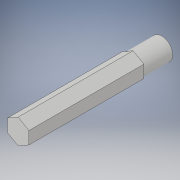
# Autodesk Inventor part: Sanded Hex Rod
Saved by Autodesk Inventor 2018 (Build 220112000, 112)
## iProperties
Created: 2019-01-13
Part Number: Sanded Hex Rod
Material: Generic
Document SubType Name: Modeling
Designer: Gabriel
Density: 1 g/cm^3
Appearance: Default
Author: Gabriel
Autodesk Inventor part; units mm, degrees
ref_plane "YZ Plane" through (0, 0, 0) normal (1, 0, 0) x (0, 1, 0)
ref_plane "XZ Plane" through (0, 0, 0) normal (0, 1, 0) x (-1, 0, 0)
ref_plane "XY Plane" through (0, 0, 0) normal (0, 0, 1) x (1, 0, 0)
sketch "Sketch1" plane through (0, 0, 0) normal (0, 0, 1) x (1, 0, 0)
  line L0 (-16.4487, 14.1051) -> (-9.6381, 18.058)
  line L1 (-16.4487, 14.1051) -> (-18.8393, 18.2241)
  line L2 (-18.8393, 12.7176) -> (-23.6081, 15.4709)
  line L3 (-23.6081, 15.4709) -> (-23.6081, 20.9774)
  line L4 (-23.6081, 20.9774) -> (-18.8393, 23.7306)
  line L5 (-18.8393, 23.7306) -> (-14.0705, 20.9774)
  line L6 (-14.0705, 20.9774) -> (-14.0705, 15.4709)
  line L7 (-14.0705, 15.4709) -> (-18.8393, 12.7176)
  dimension "d5" = 4.7625
  constraints: 16 end point, 1 coincident, 13 other
  measures "d5" distance of L0.start L1.end
extrude "Extrusion1" add sketch "Sketch1" along normal blind 50.8
sketch "Sketch3" plane through (0, 0, 0) normal (0, 0, -1) x (-1, 0, 0)
  line L0 (23.6081, 15.4709) -> (18.8393, 12.7176) projected
  line L1 (18.8393, 12.7176) -> (18.8393, 18.2241)
  circle A0 centre (18.8393, 18.2241) radius 4.7688
  point P0 (0, 0)
  constraints: 2 end point, 1 centre point, 1 coincident, 1 tangent, 1 vertical
extrude "Extrusion3" add sketch "Sketch3" along normal blind 12.7 contours A0
body "Solid1"
